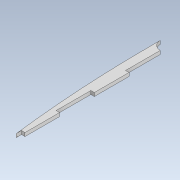
# Autodesk Inventor part: aileron_static
Saved by Autodesk Inventor 2020 (Build 240168000, 168)
## iProperties
Created: 2020-09-10
Part Number: aileron_static
Material: Generic
Document SubType Name: Modeling
Designer: Admin
Density: 1 g/cm^3
Appearance: Default
Author: Admin
Autodesk Inventor part; units mm, degrees
ref_plane "YZ Plane" through (0, 0, 0) normal (1, 0, 0) x (0, 1, 0)
ref_plane "XZ Plane" through (0, 0, 0) normal (0, 1, 0) x (-1, 0, 0)
ref_plane "XY Plane" through (0, 0, 0) normal (0, 0, 1) x (1, 0, 0)
sketch "Sketch1" plane through (0, 0, 0) normal (0, 1, 0) x (-1, 0, 0)
  line L0 (0, 0) -> (0, -83)
  arc A0 (5, -88) -> (0, -83) centre (0, -88) ccw
  line L1 (5, -83) -> (5, -88)
  arc A1 (5, -83) -> (0, 0) centre (-686.4, -83) ccw
  dimension "d3" = 0
  dimension "d4" = 0
  dimension "d5" = 5
  constraints: 4 end point, 4 point on circle, 2 centre point, 1 coincident
  measures "d3" distance from line of A0.centre L0
  measures "d4" vertical distance of A0.centre L1.end
  measures "d5" radius of A0
extrude "Extrusion1" add sketch "Sketch1" along normal blind 2
sketch "Sketch3" plane through (0, 0, 0) normal (1, 0, 0) x (0, 0, -1)
  line L0 (3, 2) -> (23, 2)
  line L1 (23, 2) -> (23, 0)
  line L2 (23, 0) -> (3, 0)
  line L3 (3, 0) -> (3, 2)
  line L4 (0, 0) -> (0, 2) projected
  line L5 (0, 0) -> (83, 0) projected
  dimension "d15" = 20
  dimension "d16" = 2
  dimension "d17" = 3
  constraints: 8 end point, 2 parallel, 1 horizontal, 1 perpendicular, 1 point on line
  measures "d15" distance of L0.start L0.end
  measures "d16" distance of L2.end L0.start
  measures "d17" distance between parallel lines of L3 L4
extrude "Extrusion3" add sketch "Sketch3" along normal blind 2
pattern_linear "Rectangular Pattern2" count 2 spacing 40 along (0, 0, -1) of "Extrusion3"
body "Solid1"
